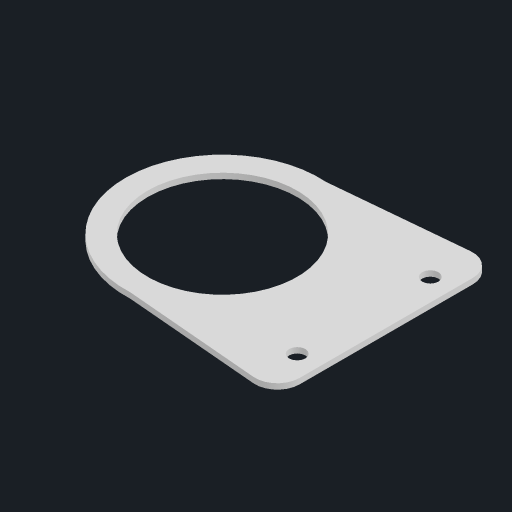
# Autodesk Inventor part: tankHolder
Saved by Autodesk Inventor 2024.2 (Build 282272000, 272)
## iProperties
Created: 2024-01-16
Part Number: tankHolder
Material: Generic
Document SubType Name: Sheet Metal
Designer: reima
Density: 1 g/cm^3
Sheet Metal Rule: Default
Appearance: Default
Author: reima
Autodesk Inventor part; units mm, degrees
ref_plane "YZ Plane" through (0, 0, 0) normal (1, 0, 0) x (0, 1, 0)
ref_plane "XZ Plane" through (0, 0, 0) normal (0, 1, 0) x (-1, 0, 0)
ref_plane "XY Plane" through (0, 0, 0) normal (0, 0, 1) x (1, 0, 0)
sketch "Sketch1" plane through (0, 0, 0) normal (0, 1, 0) x (-1, 0, 0)
  circle A0 centre (0, 0) radius 21.3995
  circle A1 centre (0, 0) radius 27.7495
  line L0 (-46.8122, -23.6104) -> (-46.8122, 23.6104)
  circle A2 centre (-40.4622, -19.05) radius 2.3368
  circle A3 centre (-40.4622, 19.05) radius 2.3368
  line L1 (-40.4622, 19.05) -> (-40.4622, -19.05) construction
  line L2 (-39.9143, 31.0559) -> (-1.3558, 27.7164)
  line L3 (-39.8743, -31.2016) -> (-1.9834, -27.6785)
  line L4 (-46.8122, 24.7296) -> (-46.8122, 23.6104)
  line L5 (-46.8122, -23.6104) -> (-46.8122, -24.8789)
  arc A4 (-39.9143, 31.0559) -> (-46.8122, 24.7296) centre (-40.4622, 24.7296) ccw
  arc A5 (-46.8122, -24.8789) -> (-39.8743, -31.2016) centre (-40.4622, -24.8789) ccw
  point P0 (-46.8122, -31.8467)
  point P1 (-46.8122, 31.6533)
  point P2 (-46.8122, 0)
  point P3 (1.3558, 27.7164)
  point P4 (1.9834, -27.6785)
  point P5 (-40.4622, 0)
  dimension "d0" = 42.799
  dimension "d1" = 6.35
  dimension "d2" = 63.5
  dimension "d4" = 0
  dimension "d8" = 4.6736
  dimension "d9" = 4.6736
  dimension "d10" = 38.1
  dimension "d11" = 6.35
  dimension "d12" = 0
  dimension "d17" = 6.35
  dimension "d18" = 6.35
  dimension "d19" = 40.4622
  dimension "d20" = 10.262
  dimension "d21" = 84.688
  dimension "d22" = 27.376
  dimension "d23" = 0.3673
  dimension "d24" = 54.8478
  dimension "d25" = 55.219
  measures "d0" diameter of A0
  measures "d1" radial gap between concentric circles of A0 A1
  measures "d2" distance of point (-46.812, -31.847) point (-46.812, 31.653)
  measures "d4" vertical distance of point (0, 0) point (-46.812, 0)
  measures "d8" diameter of A2
  measures "d9" diameter of A3
  measures "d10" distance of L1.end L1.start
  measures "d11" distance from line of L0 L1.start
  measures "d12" vertical distance of point (-46.812, 0) point (-40.462, 0)
  measures "d17" radius of A4
  measures "d18" radius of A5
  measures "d19" horizontal distance of L1.end A0.centre
  measures "d20" angle of L2 L3
  measures "d21" angle of L3 L1
  measures "d22" distance from line of point (0, 0) L3
  measures "d23" distance from line of A1.end L3
  measures "d24" distance from line of A1.start L3
  measures "d25" distance from line of L0.end L3
extrude "Plate1" add sketch "Sketch1" along normal blind 1.5875
equation "\"d13\" = Thickness"
equation "\"BendRadius\" = Thickness"
equation "\"BendReliefWidth\" = Thickness"
equation "\"BendReliefDepth\" = 0.5 * Thickness"
equation "\"CornerReliefSize\" = 4 * Thickness"
equation "\"MinimumRemnant\" = 2 * Thickness"
equation "\"TransitionRadius\" = BendRadius"
equation "\"JacobiRadiusSize\" = BendRadius"
equation "\"GapSize\" = Thickness"
equation "\"Thickness\" = 1.5875"
body "Solid1"
